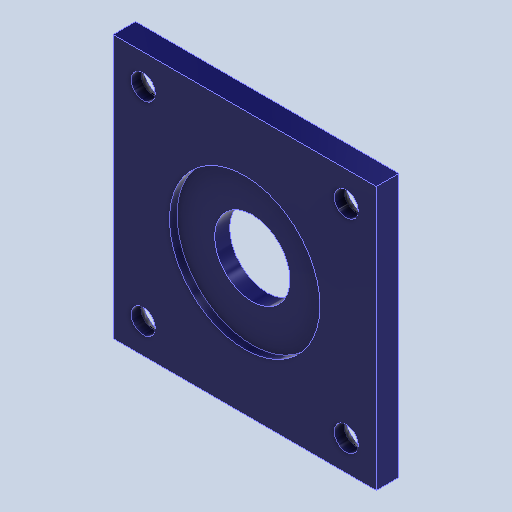
# Autodesk Inventor part: Shaft cap
Saved by Autodesk Inventor 2022 (Build 260153000, 153)
## iProperties
Created: 2022-02-10
Part Number: Shaft cap
Material: PET Plastic
Document SubType Name: Modeling
Designer: br4ch
Density: 1.541 g/cm^3
Appearance: Polycarbonate - Clear
Author: br4ch
Autodesk Inventor part; units mm, degrees
ref_plane "YZ Plane" through (0, 0, 0) normal (1, 0, 0) x (0, 1, 0)
ref_plane "XZ Plane" through (0, 0, 0) normal (0, 1, 0) x (-1, 0, 0)
ref_plane "XY Plane" through (0, 0, 0) normal (0, 0, 1) x (1, 0, 0)
sketch "Sketch1" plane through (0, 0, 0) normal (0, 0, 1) x (1, 0, 0)
  line L0 (17.5, -17.5) -> (-17.5, -17.5)
  line L1 (-17.5, -17.5) -> (-17.5, 17.5)
  line L2 (-17.5, 17.5) -> (17.5, 17.5)
  line L3 (17.5, 17.5) -> (17.5, -17.5)
  line L4 (17.5, -17.5) -> (-17.5, 17.5) construction
  line L5 (-17.5, -17.5) -> (17.5, 17.5) construction
  circle A0 centre (-13.4987, -13.4987) radius 1.5
  circle A1 centre (13.4987, -13.4987) radius 1.5
  circle A2 centre (13.4987, 13.4987) radius 1.5
  circle A3 centre (-13.4987, 13.4987) radius 1.5
  circle A4 centre (0, 0) radius 5
  circle A5 centre (0, 0) radius 10
  dimension "d0" = 35
  dimension "d1" = 35
  dimension "d3" = 3
  dimension "d6" = 360
  dimension "d8" = 10
  dimension "d9" = 20
  constraints: 12 end point, 6 centre point, 2 coincident, 2 midpoint, 2 parallel, 1 horizontal, 1 perpendicular, 1 point on line, 9 other
  measures "d0" distance of L1.end L2.end
  measures "d1" distance of L0.end L1.end
  measures "d3" diameter of A0
  measures "d8" diameter of A4
  measures "d9" diameter of A5
extrude "Extrusion1" add sketch "Sketch1" against normal blind 3 contours L0 L1 L2 L3 | A0 | A1 | A2 | A3 | A5
extrude "Extrusion2" cut sketch "Sketch1" against normal blind 1 contours A5
sketch "Sketch2" plane through (0, 0, -3) normal (0, 0, -1) x (-1, 0, 0)
  circle A0 centre (13.4987, 13.4987) radius 1.5 projected
  circle A1 centre (-13.4987, 13.4987) radius 1.5 projected
  circle A2 centre (-13.4987, -13.4987) radius 1.5 projected
  circle A3 centre (13.4987, -13.4987) radius 1.5 projected
  point P0 (0, 0)
hole "Hole2" at (13.4987, 13.4987, -3) at (-13.4987, 13.4987, -3) at (-13.4987, -13.4987, -3) at (13.4987, -13.4987, -3) direction (0, 0, 1) diameter 3.2 depth 3 tip angle 118 countersink diameter 6.6 countersink angle 90
body "Solid1"
